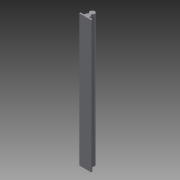
# Autodesk Inventor part: sbr20_500mm
Saved by Autodesk Inventor 2014 (Build 180170000, 170)
## iProperties
Created: 2014-08-18
Part Number: sbr20_500mm
Material: Generic
Document SubType Name: Modeling
Designer: Matthew
Density: 1 g/cm^3
Appearance: Default
Mass: 349.21 g
Surface Area: 824.464 cm^2
Volume: 349.21 cm^3
Author: Matthew
Autodesk Inventor part; units mm, degrees
ref_plane "YZ Plane" through (0, 0, 0) normal (1, 0, 0) x (0, 1, 0)
ref_plane "XZ Plane" through (0, 0, 0) normal (0, 1, 0) x (-1, 0, 0)
ref_plane "XY Plane" through (0, 0, 0) normal (0, 0, 1) x (1, 0, 0)
sketch "Sketch1" plane through (0, 0, 0) normal (0, 0, 1) x (1, 0, 0)
  line L0 (-22.5, 0) -> (22.5, 0)
  line L1 (22.5, 0) -> (22.5, 5)
  line L2 (-22.5, 0) -> (-22.5, 5)
  line L3 (-22.5, 5) -> (-9.5, 5)
  line L4 (22.5, 5) -> (9.5, 5)
  line L5 (-9.5, 5) -> (-9.5, 10)
  line L6 (9.5, 5) -> (9.5, 10)
  arc A0 (4, 18.6042) -> (-4, 18.6042) centre (0, 27) ccw
  line L7 (4, 18.6042) -> (8.9676, 10)
  line L8 (-4, 18.6042) -> (-8.9676, 10)
  line L9 (-9.5, 10) -> (9.5, 10) construction
  line L10 (-8.9676, 10) -> (-9.5, 10) construction
  line L11 (-8.9676, 10) -> (-9.5, 10)
  line L12 (8.9676, 10) -> (9.5, 10)
  line L13 (-11.4601, 5) -> (-11.4601, 0) construction
  line L14 (-16.9601, 5) -> (-16.9601, 0) construction
  line L15 (13.0399, 5) -> (13.0399, 0) construction
  line L16 (18.5399, 5) -> (18.5399, 0) construction
  arc A1 (-4, 18.6042) -> (4, 18.6042) centre (0, 27) ccw construction
  point P0 (0, 0)
  point P1 (0, 0)
  point P2 (0, 17.7)
  point P3 (15.7899, 5)
  point P4 (-14.2101, 5)
  dimension "B" = 45
  dimension "t" = 5
  dimension "d2" = 5
  dimension "dimensionf" = 19
  dimension "d4" = 13
  dimension "Y" = 10
  dimension "d6" = 5
  dimension "d" = 18.6
  dimension "e" = 22.5
  dimension "dimensionH" = 17.7
  dimension "dimensionh" = 27
  dimension "x" = 8
  dimension "d16" = 4
  dimension "dimensionc" = 30
  dimension "d21" = 6.7101
  dimension "s1" = 5.5
  dimension "d23" = 5.5
  dimension "d24" = 2.75
  dimension "d25" = 2.75
  constraints: 34 end point, 10 point on line, 6 perpendicular, 4 collinear, 4 point on circle, 3 parallel, 2 centre point, 1 coincident, 1 horizontal, 1 midpoint, 1 vertical alignment
  measures "B" distance of L0.start L0.end
  measures "t" distance of L0.start L2.end
  measures "d2" distance of L0.end L1.end
  measures "dimensionf" distance of L4.end L3.end
  measures "d4" distance of L2.end L3.end
  measures "Y" distance from line of L0 L5.end
  measures "d6" distance of L4.end L6.end
  measures "d" diameter of A0
  measures "e" distance from line of L2 A0.centre
  measures "dimensionH" distance from line of L0 point (0, 17.7)
  measures "dimensionh" distance from line of L0 A0.centre
  measures "x" distance of L7.start L8.start
  measures "d16" horizontal distance of point (0, 17.7) L7.start
  measures "dimensionc" distance of point (-14.21, 5) point (15.79, 5)
  measures "d21" distance from line of L1 point (15.79, 5)
  measures "s1" distance between parallel lines of L14 L13
  measures "d23" distance between parallel lines of L16 L15
  measures "d24" distance from line of L15 point (15.79, 5)
  measures "d25" distance from line of point (-14.21, 5) L13
extrude "Extrusion1" add sketch "Sketch1" along normal blind 500
equation "\"d2\" = t"
equation "\"d16\" = 0.5 * x"
body "Solid1"
